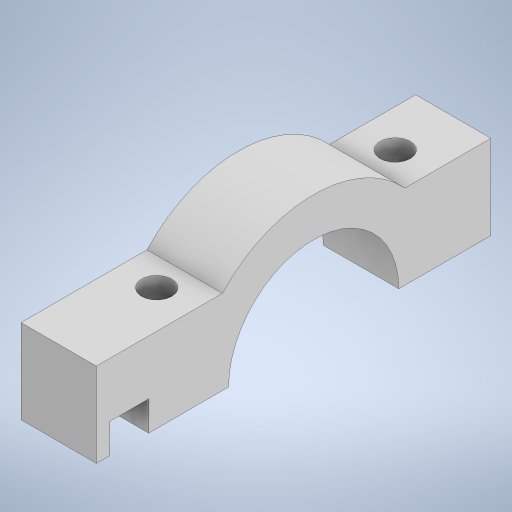
# Autodesk Inventor part: Lagerhalter2
Saved by Autodesk Inventor 2023 (Build 270158000, 158)
## iProperties
Created: 2022-05-03
Part Number: Lagerhalter2
Material: Generisch
Document SubType Name: Modeling
Designer: trist
Density: 1 g/cm^3
Appearance: Vorgabe
Author: trist
Autodesk Inventor part; units mm, degrees
ref_plane "YZ Plane" through (0, 0, 0) normal (1, 0, 0) x (0, 1, 0)
ref_plane "XZ Plane" through (0, 0, 0) normal (0, 1, 0) x (-1, 0, 0)
ref_plane "XY Plane" through (0, 0, 0) normal (0, 0, 1) x (1, 0, 0)
sketch "Skizze10" plane through (0, 0, 0) normal (1, 0, 0) x (0, 1, 0)
  arc A0 (0, -9.6) -> (0, 9.6) centre (0, 0) ccw
  line L0 (0, 0) -> (0, -20)
  line L1 (0, 0) -> (0, 24.5)
  line L2 (-2.8, 0) -> (16.8, 0) projected
  line L3 (0, 24.5) -> (9.5, 24.5)
  line L4 (9.5, 24.5) -> (9.5, 10.2835)
  arc A1 (9.5, -10.2835) -> (9.5, 10.2835) centre (0, 0) ccw
  line L5 (9.5, -10.2835) -> (9.5, -20)
  line L6 (0, -20) -> (9.5, -20)
  point P0 (0, 9.6)
  dimension "d79" = 9.6
  dimension "d80" = 20
  dimension "d81" = 24.5
  dimension "d84" = 9.5
  dimension "d85" = 14
  constraints: 12 end point, 4 point on circle, 3 vertical, 2 centre point, 2 coincident, 2 horizontal, 1 perpendicular, 1 vertical alignment
  measures "d79" radius of A0
  measures "d80" distance of L0.start L0.end
  measures "d81" distance of L0.start L1.end
  measures "d84" distance of L0.end L5.end
  measures "d85" radius of A1
extrude "Extrusion9" add sketch "Skizze10" along normal mid plane 8.5 contours A0 L2 A1 L5 L6 L0 | A0 L1 L3 L4 A1 L2
sketch "Skizze11" plane through (0, 0, 0) normal (0, 1, 0) x (-1, 0, 0)
  circle A0 centre (0, -13.45) radius 1.7
  circle A1 centre (0, 13.45) radius 1.7
  line L0 (-4.25, -20) -> (-4.25, -10.2835) projected
  line L1 (0, -27.03) -> (0, 22.18) projected
  point P0 (0, 0)
  dimension "d88" = 13.45
  dimension "d89" = 13.45
  dimension "d90" = 3.4
  dimension "d91" = 3.4
  constraints: 2 centre point, 2 point on line
  measures "d88" distance of point (0, 0) A1.centre
  measures "d89" distance of point (0, 0) A0.centre
  measures "d90" diameter of A1
  measures "d91" diameter of A0
extrude "Extrusion10" cut sketch "Skizze11" along normal through all
sketch "Skizze12" plane through (0, 0, 0) normal (0, 1, 0) x (-1, 0, 0)
  line L0 (1.05, 23) -> (-4.25, 23)
  line L1 (-4.25, 18.6) -> (1.05, 18.6)
  line L2 (2.11, 0) -> (-5.31, 0) projected
  line L3 (-4.25, 10.2835) -> (-4.25, 24.5) projected
  line L4 (1.05, 23) -> (1.05, 18.6)
  point P0 (0, 0)
  dimension "d94" = 4.4
  dimension "d95" = 5.3
  dimension "d99" = 18.6
  constraints: 6 end point, 2 point on line, 1 horizontal, 1 parallel, 1 perpendicular
  measures "d94" distance of L0.end L1.start
  measures "d95" distance of L0.start L0.end
  measures "d99" distance between parallel lines of L2 L1
extrude "Extrusion11" cut sketch "Skizze12" along normal blind 3.35
